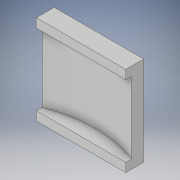
# Autodesk Inventor part: 00_cylindrical_lens_mould
Saved by Autodesk Inventor 2019 (Build 230136000, 136)
## iProperties
Created: 2021-01-25
Part Number: 00_cylindrical_lens_mould
Material: Generic
Document SubType Name: Modeling
Designer: marsikovabarbora
Density: 1 g/cm^3
Appearance: Default
Author: marsikovabarbora
Autodesk Inventor part; units mm, degrees
ref_plane "YZ Plane" through (0, 0, 0) normal (1, 0, 0) x (0, 1, 0)
ref_plane "XZ Plane" through (0, 0, 0) normal (0, 1, 0) x (-1, 0, 0)
sketch "Sketch1" plane through (0, 0, 0) normal (0, 0, 1) x (1, 0, 0)
  line L0 (-17.5, 0) -> (17.5, 0) construction
  line L1 (0, -17.5) -> (0, 17.5) construction
  line L2 (-12.5, -12.5) -> (12.5, -12.5)
  line L3 (12.5, -12.5) -> (12.5, 12.5)
  line L4 (12.5, 12.5) -> (-12.5, 12.5)
  line L5 (-12.5, 12.5) -> (-12.5, -12.5)
  line L6 (-12.5, -12.5) -> (12.5, 12.5) construction
  line L7 (12.5, -12.5) -> (-12.5, 12.5) construction
  point P0 (0, 0)
  dimension "d0" = 25
  dimension "d1" = 25
  constraints: 12 end point, 2 midpoint, 2 parallel, 1 horizontal, 1 perpendicular
  measures "d0" distance of L2.end L3.end
  measures "d1" distance of L3.end L4.end
extrude "Extrusion1" add sketch "Sketch1" along normal blind 5
ref_plane "Work Plane1" through (-12.5, 10, 0) normal (0, 1, 0) x (1, 0, 0)
sketch "Sketch2" plane through (-12.5, 10, 0) normal (0, 1, 0) x (1, 0, 0)
  line L0 (25, 0) -> (0, 0) construction
  line L1 (0, 0) -> (0, -5) construction
  line L2 (25, -5) -> (0, -5) construction
  line L3 (25, 0) -> (25, -5) construction
  line L4 (12.5, 0) -> (12.5, -5) construction
  circle A0 centre (12.5, -35.334) radius 34.284
  line L5 (-3.4763, -5) -> (28.4763, -5)
  dimension "d5" = 68.568
  dimension "d6" = 30.334
  constraints: 4 end point, 2 point on circle, 1 centre point, 1 collinear, 1 horizontal, 1 midpoint, 1 point on line
  measures "d5" diameter of A0
  measures "d6" distance from line of A0.centre L5
extrude "Extrusion2" cut sketch "Sketch2" against normal blind 20
body "Solid1"
